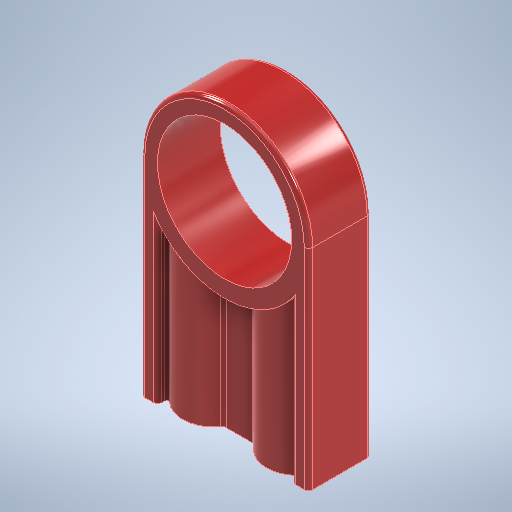
# Autodesk Inventor part: Steering Support
Saved by Autodesk Inventor 2025.2 (Build 292293000, 293)
## iProperties
Created: 2025-02-04
Part Number: Steering Support
Material: Generic
Document SubType Name: Modeling
Designer: eason
Density: 1 g/cm^3
Appearance: Red
Author: eason
Autodesk Inventor part; units mm, degrees
ref_plane "YZ Plane" through (0, 0, 0) normal (1, 0, 0) x (0, 1, 0)
ref_plane "XZ Plane" through (0, 0, 0) normal (0, 1, 0) x (-1, 0, 0)
ref_plane "XY Plane" through (0, 0, 0) normal (0, 0, 1) x (1, 0, 0)
sketch "Sketch1" plane through (0, 0, 0) normal (0, 0, 1) x (1, 0, 0)
  circle A0 centre (0, 0) radius 16
  arc A1 (20, 0) -> (-20, 0) centre (0, 0) ccw
  line L0 (20, 0) -> (20, -50)
  line L1 (20, -50) -> (-20, -50)
  line L2 (-20, -50) -> (-20, 0)
  line L3 (-28, 0) -> (28, 0) projected
  circle A2 centre (0, 0) radius 20
  point P0 (-20, 0)
  point P1 (20, 0)
  point P2 (20, 0)
  point P3 (-20, 0)
  dimension "d0" = 32
  dimension "d1" = 40
  dimension "d2" = 50
  constraints: 6 end point, 3 centre point, 3 coincident, 2 point on circle, 2 point on line, 2 tangent, 1 concentric, 1 parallel
  measures "d0" diameter of A0
  measures "d1" diameter of A1
  measures "d2" distance between parallel lines of L3 L1
extrude "Extrusion1" add sketch "Sketch1" along normal blind 15 contours L3 A2 A0 | A0 L3 A1
extrude "Extrusion3" add sketch "Sketch1" along normal blind 15 contours L0 L1 L2 A2
sketch "Sketch4" plane through (-20, -50, 0) normal (0, -1, 0) x (1, 0, 0)
  circle A0 centre (10, 7.5) radius 4
  circle A1 centre (10, 7.5) radius 7.5
  line L0 (0, 15) -> (40, 15) projected
  line L1 (0, 0) -> (40, 0) projected
  line L2 (0, 0) -> (0, 15) projected
  line L3 (20, 15) -> (20, 0) construction
  line L4 (4, 15) -> (4, 12)
  line L5 (4, 3) -> (4, 0)
  circle A2 centre (30, 7.5) radius 4
  circle A3 centre (30, 7.5) radius 7.5
  line L6 (36, 15) -> (36, 12)
  line L7 (36, 3) -> (36, 0)
  line L8 (16.3443, 11.5) -> (23.6557, 11.5)
  line L9 (16.3443, 3.5) -> (23.6557, 3.5)
  point P0 (20, 0)
  point P1 (4, 13.5)
  point P2 (10, 0)
  point P3 (30, 0)
  point P4 (36, 0)
  point P5 (30, 15)
  point P6 (10, 15)
  dimension "d25" = 8
  dimension "d26" = 10
  dimension "d27" = 4
  dimension "d29" = 15
  constraints: 14 end point, 8 point on circle, 6 point on line, 6 symmetric about line, 4 centre point, 4 tangent, 3 midpoint, 2 coincident, 1 horizontal, 1 parallel, 1 vertical, 2 other
  measures "d25" diameter of A0
  measures "d26" distance from line of L2 A0.centre
  measures "d27" distance from line of point (4, 13.5) L2
  measures "d29" distance between parallel lines of L1 L0
extrude "Extrusion4" cut sketch "Sketch4" against normal up to surface contours A1 L0 A3 L8 | L9 A3 L1 A1 | A1 L4 L0 | L1 L5 A1 | L0 L6 A3 | A3 L7 L1 round surface about axis through (0, 0, 0) along (0, 0, 1) radius 20 far side no
extrude "Extrusion5" cut sketch "Sketch4" against normal up to surface contours A0 | A2 round surface about axis through (0, 0, -41.9777) along (0, 0, 1) radius 20 far side no
thread "Thread3" size "M8x1.25" class "6H" standard "ANSI Metric M Profile" full length
thread "Thread4" size "M8x1.25" class "6H" standard "ANSI Metric M Profile" full length
fillet "Fillet2" radius 1 14 edges at (0, 20, 15) (-20, -25, 15) (20, -25, 15) (0, 20, 0) (-20, -25, 0) (20, -25, 0) (-16, -31, 15) (16, -31, 15) (-16, -31, 0) (16, -31, 0) (-3.6557, -34.8315, 11.5) (3.6557, -34.8315, 11.5) (-3.6557, -34.8315, 3.5) (3.6557, -34.8315, 3.5)
fillet "Fillet3" radius 0.5 4 edges at (-16, -31, 12) (16, -31, 12) (16, -31, 3) (-16, -31, 3)
body "Solid1"
